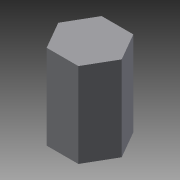
# Autodesk Inventor part: 129_3
Saved by Autodesk Inventor 2014 (Build 180170000, 170)
## iProperties
Created: 2017-04-22
Part Number: 129_3
Material: Generic
Document SubType Name: Modeling
Designer: Andy
Density: 1 g/cm^3
Appearance: Default
Author: Andy
Autodesk Inventor part; units mm, degrees
ref_plane "YZ Plane" through (0, 0, 0) normal (1, 0, 0) x (0, 1, 0)
ref_plane "XZ Plane" through (0, 0, 0) normal (0, 1, 0) x (-1, 0, 0)
ref_plane "XY Plane" through (0, 0, 0) normal (0, 0, 1) x (1, 0, 0)
sketch "Sketch1" plane through (0, 0, 0) normal (0, 1, 0) x (-1, 0, 0)
  line L0 (-3.7437, 0) -> (-1.8719, 3.2422)
  line L1 (-1.8719, 3.2422) -> (1.8719, 3.2422)
  line L2 (1.8719, 3.2422) -> (3.7437, 0)
  line L3 (3.7437, 0) -> (1.8719, -3.2422)
  line L4 (1.8719, -3.2422) -> (-1.8719, -3.2422)
  line L5 (-1.8719, -3.2422) -> (-3.7437, 0)
  point P0 (0, 0)
  point P1 (0, 0)
  constraints: 12 end point, 1 coincident, 13 other
extrude "Extrusion1" add sketch "Sketch1" along normal blind 10
body "Solid1"
